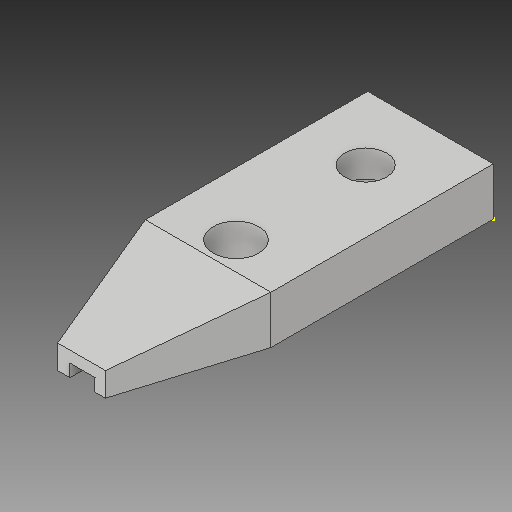
# Autodesk Inventor part: HeadbarClampBottom
Saved by Autodesk Inventor 2019 (Build 230136000, 136)
## iProperties
Created: 2015-12-02
Part Number: HeadbarClampBottom
Material: Generic
Document SubType Name: Modeling
Designer: Vervaeke-Lab
Density: 1 g/cm^3
Appearance: Default
Author: Vervaeke-Lab
Autodesk Inventor part; units mm, degrees
ref_plane "YZ Plane" through (0, 0, 0) normal (1, 0, 0) x (0, 1, 0)
ref_plane "XZ Plane" through (0, 0, 0) normal (0, 1, 0) x (-1, 0, 0)
ref_plane "XY Plane" through (0, 0, 0) normal (0, 0, 1) x (1, 0, 0)
sketch "Sketch1" plane through (0, 0, 0) normal (0, 1, 0) x (-1, 0, 0)
  line L0 (0, 0) -> (12.6, 0)
  line L1 (12.6, 0) -> (12.6, 22.3)
  line L2 (0, 0) -> (0, 22.3)
  line L3 (0, 22.3) -> (3.9, 35)
  line L4 (3.9, 35) -> (8.7, 35)
  line L5 (8.7, 35) -> (12.6, 22.3)
  point P0 (6.3, 6.5)
  dimension "d4" = 22.3
  dimension "d5" = 4.8
  constraints: 12 end point, 1 horizontal
  measures "d4" distance of L0.end L1.end
  measures "d5" distance of L3.end L4.end
extrude "Extrusion1" add sketch "Sketch1" along normal blind 4.8
sketch "Sketch2" plane through (0, 0, 0) normal (0, -1, 0) x (1, 0, 0)
  point P0 (0, 0)
  point P1 (-6.3, 6.5)
hole "Hole1" at (-6.3, 0, 6.5) direction (0, 1, 0) diameter 4.2 depth 8 tip angle 118 countersink diameter 8.4 countersink angle 90
sketch "Sketch3" plane through (0, 0, 0) normal (0, -1, 0) x (1, 0, 0)
  circle A0 centre (-6.3, 19.5) radius 2.3
  point P0 (0, 0)
  dimension "d13" = 4.6
  constraints: 1 centre point, 1 coincident
  measures "d13" diameter of A0
extrude "Extrusion2" cut sketch "Sketch3" against normal through all
sketch "Sketch4" plane through (0, 0, 0) normal (1, 0, 0) x (0, 1, 0)
  line L0 (0, 35) -> (4.8, 35) projected
  line L1 (0, 22.3) -> (4.8, 22.3) projected
  line L2 (4.8, 22.3) -> (2.4, 35)
  line L3 (4.8, 35) -> (4.8, 22.3) projected
  line L4 (2.4, 35) -> (4.8, 35)
  line L5 (4.8, 35) -> (4.8, 22.3)
  point P0 (0, 0)
  constraints: 6 end point, 1 collinear, 1 horizontal, 1 midpoint
extrude "Extrusion3" cut sketch "Sketch4" against normal through all
sketch "Sketch5" plane through (0, 0, 0) normal (1, 0, 0) x (0, 1, 0)
  point P0 (0, 0)
sketch "Sketch6" plane through (0, 0, 0) normal (0, -1, 0) x (1, 0, 0)
  line L0 (-8.7, 35) -> (-3.9, 35) projected
  line L1 (-4.9584, 35) -> (-7.4584, 35)
  line L2 (-7.4584, 35) -> (-7.4584, 33)
  line L3 (-7.4584, 33) -> (-4.9584, 33)
  line L4 (-4.9584, 33) -> (-4.9584, 35)
  point P0 (0, 0)
  point P1 (-6.3, 35)
  dimension "d18" = 2.5
  dimension "d19" = 2
  constraints: 8 end point, 2 parallel, 1 horizontal, 1 midpoint, 1 perpendicular, 1 point on line
  measures "d18" distance of L3.end L2.end
  measures "d19" distance of L2.end L1.end
extrude "Extrusion4" cut sketch "Sketch6" against normal blind 1.27
body "Solid1"
